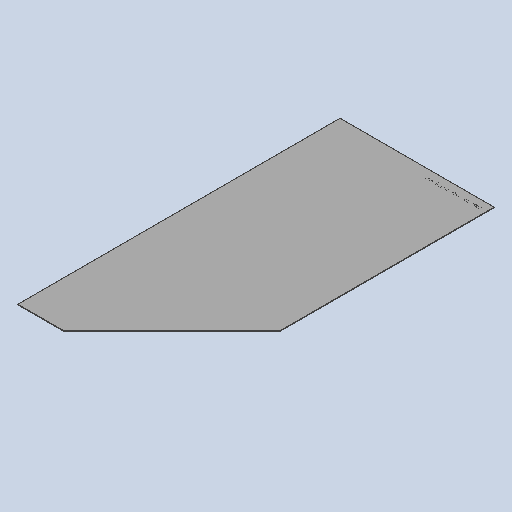
# Autodesk Inventor part: TRM 015 left board main
Saved by Autodesk Inventor 2025 (Build 290162010, 162A)
## iProperties
Created: 2024-08-07
Part Number: TRM 015 left board main
Material: AISI 304
Document SubType Name: Sheet Metal
Designer: pokla
Density: 8.02768 g/cm^3
Flat Pattern Width: 50.2 cm
Flat Pattern Length: 105 cm
Flat Pattern Area: 5271 cm^2
Sheet Metal Rule: AISI304 2mm Die16
Sheet Metal Width: 502,000 mm
Sheet Metal Length: 1050,000 mm
Sheet Metal Area: 527100,000 mm^2
Appearance: Default
Stock Number: ТРМ 015 левый борт основное
Author: pokla
Autodesk Inventor part; units mm, degrees
ref_plane "YZ Plane" through (0, 0, 0) normal (1, 0, 0) x (0, 1, 0)
ref_plane "XZ Plane" through (0, 0, 0) normal (0, 1, 0) x (-1, 0, 0)
ref_plane "XY Plane" through (0, 0, 0) normal (0, 0, 1) x (1, 0, 0)
sketch "Sketch1" plane through (0, 0, 0) normal (0, 0, 1) x (1, 0, 0)
  line L0 (-251, -525) -> (251, -525)
  line L1 (251, -525) -> (251, 525)
  line L2 (251, 525) -> (-251, 525)
  line L3 (-251, 525) -> (-251, -525)
  line L4 (-251, -525) -> (251, 525) construction
  line L5 (251, -525) -> (-251, 525) construction
  line L6 (-101, -525) -> (251, -173)
  point P0 (0, 0)
  dimension "d0" = 502
  dimension "d1" = 1050
  dimension "d12" = 698
  dimension "d13" = 150
  measures "d0" distance of L2.end L1.end
  measures "d1" distance of L1.end L0.end
  measures "d12" distance of L6.end L1.end
  measures "d13" distance of L6.start L0.start
extrude "Plate1" add sketch "Sketch1" along normal blind 2 contours L3 L2 L1 L6 L0
sketch "Sketch2" plane through (0, 0, 0) normal (0, 0, -1) x (-1, 0, 0)
  line L0 (-231, 505) -> (-31, 505) construction
  line L1 (-31, 505) -> (-31, 485) construction
  line L2 (-31, 485) -> (-231, 485) construction
  line L3 (-231, 485) -> (-231, 505) construction
  line L4 (-251, 525) -> (251, 525) projected
  line L5 (-251, -173) -> (-251, 525) projected
  point P0 (0, 0)
  point P1 (-48, 100)
  point P2 (-251, -525)
  point P3 (-50, 98)
  dimension "d6" = 200
  dimension "d9" = 20
  dimension "d10" = 20
  dimension "d11" = 20
  constraints: 4 other
  measures "d6" distance of L0.start L0.end
  measures "d9" distance of L0.end L1.end
  measures "d11" length of L3
mark "Mark1"
equation "\"d2\" = Thickness"
equation "\"BendReliefWidth\" = Thickness"
equation "\"BendReliefDepth\" = 0.5 * Thickness"
equation "\"CornerReliefSize\" = 4 * Thickness"
equation "\"MinimumRemnant\" = 2 * Thickness"
equation "\"TransitionRadius\" = BendRadius"
equation "\"JacobiRadiusSize\" = BendRadius"
equation "\"GapSize\" = Thickness"
equation "\"Thickness\" = 2"
equation "\"BendRadius\" = 2.75"
body "Solid1"
